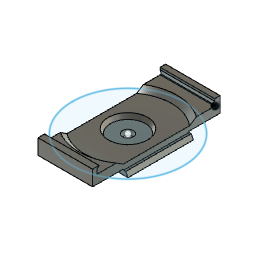
Watch Mount v1 (Autodesk Fusion 360 design; units mm, degrees)
Autodesk Fusion 360 part; units mm, degrees
note: some values were not read from the file. Set by a fixed rule: which face or edge a step refers to.
sketch "Sketch1" plane through (0, 0, 0) normal (0, 0, 1) x (1, 0, 0)
  line L0 (0, 0) -> (30, 0)
  line L1 (30, 0) -> (30, 30)
  line L2 (30, 30) -> (0, 30)
  line L3 (0, 30) -> (0, 0)
  dimension "d7" = 30
  dimension "d8" = 30
  constraint horizontal L0
  constraint vertical L1
  constraint horizontal L2
  constraint vertical L3
  constraint coincident L0.start L3.end
  measures "d7" distance of L0.start L0.end
  measures "d8" distance of L0.start L2.end
extrude "Extrude1" add sketch "Sketch1" along normal blind 2
chamfer "Chamfer1" distance 1 angle 63.4 2 edges at (30, 15, 2) (0, 15, 2) measured on face at (10, 20, 2) measured on face at (10, 20, 2)
sketch "Sketch2" plane through (0, 0, 0) normal (0, 1, 0) x (1, 0, 0)
extrude "Extrude2" add 1 faces at (10.3333, 20, 2) along direction (0, 0, 1) blind 0.5
sketch "Sketch3" plane through (0, 0, 0) normal (0, -1, 0) x (1, 0, 0)
  line L0 (1, 2) -> (0, 0.003)
  line L1 (0, 0.003) -> (0, 0)
  line L2 (0, 0) -> (30, 0)
  line L3 (30, 0) -> (30, 0.003)
  line L4 (30, 0.003) -> (29, 2)
  line L5 (29, 2) -> (29, 2.5)
  line L6 (29, 2.5) -> (1, 2.5)
  line L7 (1, 2.5) -> (1, 2)
extrude "Extrude3" add 1 faces at (10.3333, 20, 2.5) along direction (0, 0, 1) blind 2
sketch "Sketch4" plane through (0, 30, 0) normal (0, 1, 0) x (-1, 0, 0)
  line L0 (0, 0.003) -> (-1, 2)
  line L1 (-1, 2) -> (-1, 4.5)
  line L2 (-1, 4.5) -> (-29, 4.5)
  line L3 (-29, 4.5) -> (-29, 2)
  line L4 (-29, 2) -> (-30, 0.003)
  line L5 (-30, 0.003) -> (-30, 0)
  line L6 (-30, 0) -> (0, 0)
  line L7 (0, 0) -> (0, 0.003)
  line L8 (-29, 2.4884) -> (-1, 2.4884)
  line L9 (-1, 2.4884) -> (-1, 4.5)
  line L10 (-1, 4.5) -> (-29, 4.5)
  line L11 (-29, 4.5) -> (-29, 2.4884)
  constraint horizontal L8
  constraint vertical L9
  constraint horizontal L10
  constraint vertical L11
  constraint coincident L1.end L2.start
  constraint coincident L3 L8.start
sketch "Sketch5" plane through (0, 0, 0) normal (0, -1, 0) x (1, 0, 0)
sketch "Sketch6" plane through (0, 0, 0) normal (0, -1, 0) x (1, 0, 0)
  line L0 (1, 2) -> (0, 0.003)
  line L1 (0, 0.003) -> (0, 0)
  line L2 (0, 0) -> (30, 0)
  line L3 (30, 0) -> (30, 0.003)
  line L4 (30, 0.003) -> (29, 2)
  line L5 (29, 2) -> (29, 4.5)
  line L6 (29, 4.5) -> (1, 4.5)
  line L7 (1, 4.5) -> (1, 2)
  line L8 (29, 2.5089) -> (1, 2.5089)
  constraint coincident L5 L8.start
  constraint coincident L7 L8.end
  constraint perpendicular L7 L8
sketch "Sketch13" plane through (0, 0, 0) normal (0, -1, 0) x (1, 0, 0)
  line L0 (1, 2) -> (0, 0.003)
  line L1 (0, 0.003) -> (0, 0)
  line L2 (0, 0) -> (30, 0)
  line L3 (30, 0) -> (30, 0.003)
  line L4 (30, 0.003) -> (29, 2)
  line L5 (29, 2) -> (29, 4.5)
  line L6 (29, 4.5) -> (1, 4.5)
  line L7 (1, 4.5) -> (1, 2)
  line L8 (29, 2.4573) -> (1, 2.4573)
  constraint coincident L5 L8.start
  constraint coincident L7 L8.end
  constraint perpendicular L7 L8
sketch "Sketch14" plane through (15, 30, 2.25) normal (0, 1, 0) x (-1, 0, 0)
  line L0 (-14, 0.2) -> (14, 0.2)
  constraint horizontal L0
sketch "Sketch15" plane through (0, 0, 0) normal (0, -1, 0) x (1, 0, 0)
sketch "Sketch17" plane through (15, 30, 2.25) normal (0, 1, 0) x (-1, 0, 0)
sketch "Sketch18" plane through (15, 30, 2.25) normal (0, 1, 0) x (-1, 0, 0)
sketch "Sketch19" plane through (0, 0, 0) normal (0, -1, 0) x (1, 0, 0)
sketch "Sketch20" plane through (29, 0, 0) normal (1, 0, 0) x (0, 1, 0)
  line L0 (0, 2) -> (30, 2)
  line L1 (30, 2) -> (30, 4.5)
  line L2 (30, 4.5) -> (0, 4.5)
  line L3 (0, 4.5) -> (0, 2)
  line L4 (0, 2.5) -> (33.766, 2.5)
  constraint coincident L3 L4.start
  constraint perpendicular L3 L4
split_face "SplitFace3" 2 faces at (19.6667, 30, 3.6667) (19.6667, 0, 3.6667) by curves path "Sketch20" along L4
extrude "Extrude6" add sketch "Sketch4" along normal blind 12.25 contours L1 L2 L3 L8 L9 L10 L11
extrude "Extrude7" add 1 faces at (10.3333, 0, 3.1667) along direction (0, -1, 0) blind 12.25
sketch "Sketch21" plane through (0, 0, 4.5) normal (0, 0, 1) x (-1, 0, 0)
  line L0 (-1, -42.25) -> (-1, 12.25)
  line L1 (-1, 12.25) -> (-29, 12.25)
  line L2 (-29, 12.25) -> (-29, -42.25)
  line L3 (-29, -42.25) -> (-1, -42.25)
  circle A0 centre (-15, -15) radius 20 construction
  circle A1 centre (-15, -15) radius 8
  dimension "d39" = 40
  dimension "d40" = 16
  constraint concentric A0 A1
  measures "d39" diameter of A0
  measures "d40" diameter of A1
extrude "Extrude8" cut sketch "Sketch21" against normal blind 2 contours A1
chamfer "Chamfer2" distance 1 angle 63.4 1 edges at (22.4586, 12.1071, 4.5) measured on face at (14.8007, -5.8259, 4.5)
sketch "Sketch22" plane through (0, 0, 2.5) normal (0, 0, 1) x (-1, 0, 0)
  circle A0 centre (-15, -15) radius 8
  circle A1 centre (-15, -15) radius 20
  dimension "d45" = 40
  constraint concentric A0 A1
  measures "d45" diameter of A1
split_face "SplitFace4" 1 faces at (14.7758, -6.1583, 4.5) by curves path "Sketch22" along A1
extrude "Extrude9" cut 1 faces at (19.6667, 34.0833, 2.4884) along direction (0, 0, 1) blind 0.012
extrude "Extrude10" add 2 faces at (15.4695, 39.8168, 4.5) (15.4695, -9.8168, 4.5) along direction (0, 0, 1) blind 2
sketch "Sketch23" plane through (0, 0, 2.5) normal (0, 0, 1) x (-1, 0, 0)
  circle A0 centre (-15, -15) radius 8
chamfer "Chamfer3" distance 2.5 angle 38.659 2 edges at (15, -5, 6.5) (15, 35, 6.5) measured on face at (15.4695, -9.8168, 6.5) measured on face at (15.4695, 39.8168, 6.5)
sketch "Watch Diameter" plane through (0, 0, 2.5) normal (0, 0, 1) x (-1, 0, 0)
  circle A0 centre (-15, -15) radius 25.5
  dimension "d53" = 51
  measures "d53" diameter of A0
extrude "Extrude11" add 1 faces at (10.3333, 42.25, 3.8336) along direction (0, 1, 0) blind 2
extrude "Extrude12" add 1 faces at (10.3333, -12.25, 3.8333) along direction (0, -1, 0) blind 2
sketch "Sketch25" plane through (0, 0, 0) normal (0, 0, 1) x (1, 0, 0)
  line L0 (-10.8875, 42.25) -> (40.8875, 42.25)
  line L1 (40.8875, 42.25) -> (40.8875, -12.25)
  line L2 (40.8875, -12.25) -> (-10.8875, -12.25)
  line L3 (-10.8875, -12.25) -> (-10.8875, 42.25)
  line L4 (-10.8875, 42.25) -> (40.8875, -12.25) construction
  line L5 (40.8875, 42.25) -> (-10.8875, -12.25) construction
  point P0 (15, 15)
  dimension "d58" = 54.5
  constraint horizontal L0
  constraint perpendicular L0 L1
  constraint parallel L0 L2
  constraint parallel L1 L3
  constraint coincident L4 P0
  constraint coincident L5 P0
  measures "d58" distance of L0.end L1.end
split_face "SplitFace5" 2 faces at (15.5591, 41.9791, 6.5) (15.5591, -11.9791, 6.5) by curves path "Sketch25" along L3 L0 L1 L2
extrude "Extrude13" cut 1 faces at (29, -5.6213, 3.8333) along direction (-1, 0, 0) blind 1
extrude "Extrude14" cut 1 faces at (1, -5.6213, 3.8333) along direction (1, 0, 0) blind 2
extrude "Extrude15" add 2 faces at (11.3333, 42.9167, 6.5) (11.3333, -12.9167, 6.5) along direction (0, 0, 1) blind 3
sketch "Sketch26" plane through (0, -12.25, 0) normal (0, 1, 0) x (-1, 0, 0)
  line L0 (-28, 6.5) -> (-3, 6.5)
  line L1 (-3, 6.5) -> (-3, 9.5)
  line L2 (-3, 9.5) -> (-28, 9.5)
  line L3 (-28, 9.5) -> (-28, 6.5)
  line L4 (-28, 6.5) -> (-3, 6.5)
  line L5 (-3, 6.5) -> (-3, 8.5)
  line L6 (-3, 8.5) -> (-28, 8.5)
  line L7 (-28, 8.5) -> (-28, 6.5)
  dimension "d65" = 2
  constraint horizontal L4
  constraint vertical L5
  constraint horizontal L6
  constraint vertical L7
  constraint coincident L0.start L3.end
  measures "d65" distance of L0.start L6.end
extrude "Extrude16" add sketch "Sketch26" along normal blind 1 contours L1 L2 L3 L6
chamfer "Chamfer4" distance 0.996 angle 45 1 edges at (15.5, -11.25, 8.5) measured on face at (19.6667, -11.25, 9.1667)
extrude "Extrude17" add 1 faces at (11.3333, 42.25, 7.5) along direction (0, -1, 0) blind 0.5
sketch "Sketch27" plane through (0, 41.75, 0) normal (0, -1, 0) x (1, 0, 0)
  line L0 (3, 6.5) -> (28, 6.5)
  line L1 (28, 6.5) -> (28, 9.5)
  line L2 (28, 9.5) -> (3, 9.5)
  line L3 (3, 9.5) -> (3, 6.5)
sketch "Sketch28" plane through (28, 0, 0) normal (1, 0, 0) x (0, 1, 0)
  line L0 (-12.246, 8.5) -> (-11.25, 9.496)
  line L1 (-11.25, 9.496) -> (-11.25, 9.5)
  line L2 (-11.25, 9.5) -> (-14.25, 9.5)
  line L3 (-14.25, 9.5) -> (-14.25, 2.5)
  line L4 (-14.25, 2.5) -> (0, 2.5)
  line L5 (0, 2.5) -> (0, 2)
  line L6 (0, 2) -> (30, 2)
  line L7 (30, 2) -> (30, 2.5004)
  line L8 (30, 2.5004) -> (44.25, 2.5004)
  line L9 (44.25, 2.5004) -> (44.25, 9.5)
  line L10 (44.25, 9.5) -> (41.75, 9.5)
  line L11 (41.75, 9.5) -> (41.75, 6.5)
  line L12 (41.75, 6.5) -> (33.3644, 6.5)
  spline S0 degree 2 poles (30.1987, 4.5001) (31.6884, 5.4057) (33.3644, 6.5) knots 0 0 0 0.374463 0.374463 0.374463 weights 1 1.002786 1
  line L13 (30.1987, 4.5001) -> (30.1987, 4.5)
  line L14 (30.1987, 4.5) -> (-0.1987, 4.5)
  line L15 (-0.1987, 4.5) -> (-0.1987, 4.5001)
  spline S1 degree 2 poles (-3.3644, 6.5) (-1.6884, 5.4057) (-0.1987, 4.5001) knots 0 0 0 0.374463 0.374463 0.374463 weights 1 1.002786 1
  line L16 (-3.3644, 6.5) -> (-12.25, 6.5)
  line L17 (-12.25, 6.5) -> (-12.25, 8.5)
  line L18 (-12.25, 8.5) -> (-12.246, 8.5)
  line L19 (41.75, 6.5) -> (42.25, 6.5)
  dimension "d72" = 0.5
  constraint coincident L11.end L12.start
  constraint horizontal L19
  measures "d72" distance of L11.end L19.end
sketch "Sketch29" plane through (28, 0, 0) normal (1, 0, 0) x (0, 1, 0)
sketch "Sketch30" plane through (0, 0, 6.5) normal (0, 0, 1) x (-1, 0, 0)
  line L0 (-28, -41.75) -> (-3, -41.75)
  line L1 (-3, -41.75) -> (-3, -34.0329)
  arc A0 (-28, -33.3644) -> (-3, -34.0329) centre (-15, -15) ccw
  line L2 (-28, -33.3644) -> (-28, -41.75)
  line L3 (-28.0001, -42.2337) -> (-3, -42.2337)
  line L4 (-3, -42.2337) -> (-3, -41.75)
  line L5 (-3, -41.75) -> (-28.0001, -41.75)
  line L6 (-28.0001, -41.75) -> (-28.0001, -42.2337)
  constraint horizontal L3
  constraint vertical L4
  constraint horizontal L5
  constraint vertical L6
  constraint coincident L0.end L1.start
split_face "SplitFace6" 1 faces at (15.5338, 40.3307, 6.5) by curves path "Sketch30" along L4 L5 L6 L3
sketch "Sketch31" plane through (15.5, 41.75, 8) normal (0, -1, 0) x (1, 0, 0)
  line L0 (12.5, -1.5) -> (-12.5, -1.5)
  line L1 (-12.5, -1.5) -> (-12.5, 0.5)
  line L2 (-12.5, 0.5) -> (12.5, 0.5)
  line L3 (12.5, 0.5) -> (12.5, -1.5)
  dimension "d73" = 2
  constraint horizontal L0
  constraint vertical L1
  constraint horizontal L2
  constraint vertical L3
  measures "d73" distance of L0.start L2.end
extrude "Extrude18" cut sketch "Sketch31" against normal blind 0.5
chamfer "Chamfer5" distance 0.5 angle 75.96 1 edges at (15.5, 42.25, 8.5) measured on face at (11.3333, 41.9167, 8.5)
sketch "Sketch32" plane through (0, 0, 2.5) normal (0, 0, 1) x (1, 0, 0)
  circle A0 centre (15, 15) radius 2.5
  dimension "d78" = 5
  measures "d78" diameter of A0
extrude "Extrude19" cut sketch "Sketch32" against normal blind 2.5
equation "baseWidth = 30 mm"
equation "baseLength = 30 mm"
equation "baseHeight = 2 mm"
equation "baseChamfer = 1 mm"
equation "d7 = baseLength"
equation "d8 = baseWidth"
equation "d9 = baseHeight"
equation "d11 = baseChamfer"
equation "watchBaseDiameter = 40 mm"
equation "watchTopOfRailToBase = 6 mm"
equation "watchHRMheight = 2 mm"
equation "watchHRMdiameter = 16 mm"
equation "watchHRMChamfer = 1 mm"
equation "watchRailtoRail = 54.5 mm"
equation "watchRailLength = 26 mm"
equation "d35 = ( watchRailtoRail - baseWidth ) / 2"
equation "d37 = ( watchRailtoRail - baseLength ) / 2"
equation "d39 = watchBaseDiameter"
equation "d40 = watchHRMdiameter"
equation "d41 = -watchHRMheight"
equation "d45 = watchBaseDiameter"
equation "d58 = watchRailtoRail"
equation "d59 = -mm"
named bodies: "Base V1"
